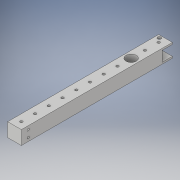
# Autodesk Inventor part: RobotArm Arm
Saved by Autodesk Inventor 2018 (Build 220112000, 112)
## iProperties
Created: 2018-01-13
Part Number: RobotArm Arm
Material: Generic
Document SubType Name: Modeling
Designer: lopez.xavier
Density: 1 g/cm^3
Appearance: Default
Author: lopez.xavier
Autodesk Inventor part; units mm, degrees
ref_plane "YZ Plane" through (0, 0, 0) normal (1, 0, 0) x (0, 1, 0)
ref_plane "XZ Plane" through (0, 0, 0) normal (0, 1, 0) x (-1, 0, 0)
ref_plane "XY Plane" through (0, 0, 0) normal (0, 0, 1) x (1, 0, 0)
sketch "Sketch1" plane through (0, 0, 0) normal (0, 0, 1) x (1, 0, 0)
  line L0 (0, 0) -> (279.4, 0)
  line L1 (279.4, 0) -> (279.4, 25.4)
  line L2 (279.4, 25.4) -> (0, 25.4)
  line L3 (0, 25.4) -> (0, 0)
  dimension "d0" = 279.4
  dimension "d1" = 25.4
  constraints: 8 end point, 2 parallel, 1 horizontal, 1 perpendicular
  measures "d0" distance of L2.end L1.end
  measures "d1" distance of L0.end L1.end
extrude "Extrusion1" add sketch "Sketch1" along normal blind 25.4
sketch "Sketch4" plane through (0, 0, 25.4) normal (0, 0, 1) x (1, 0, 0)
  circle A0 centre (12.7, 12.7) radius 2.3813
  line L0 (0, 0) -> (279.4, 0) projected
  line L1 (0, 25.4) -> (0, 0) projected
  circle A1 centre (38.1, 12.7) radius 2.3813
  circle A2 centre (63.5, 12.7) radius 2.3813
  circle A3 centre (88.9, 12.7) radius 2.3813
  circle A4 centre (114.3, 12.7) radius 2.3813
  circle A5 centre (139.7, 12.7) radius 2.3813
  circle A6 centre (165.1, 12.7) radius 2.3813
  circle A7 centre (190.5, 12.7) radius 2.3813
  circle A8 centre (215.9, 12.7) radius 2.3813
  circle A9 centre (241.3, 12.7) radius 2.3813
  circle A10 centre (266.7, 12.7) radius 2.3813
  circle A11 centre (292.1, 12.7) radius 2.3813
  circle A12 centre (317.5, 12.7) radius 2.3813
  circle A13 centre (63.5, 12.7) radius 9.525
  circle A14 centre (5.08, 6.35) radius 3.175
  dimension "d17" = 4.7625
  dimension "d18" = 12.7
  dimension "d19" = 12.7
  dimension "d22" = 25.4
  dimension "d37" = 19.05
  dimension "d46" = 6.35
  dimension "d48" = 6.35
  dimension "d49" = 58.42
  constraints: 15 centre point, 1 coincident, 1 horizontal, 24 other
  measures "d17" diameter of A0
  measures "d18" distance from line of L0 A0.centre
  measures "d19" distance from line of L1 A0.centre
  measures "d22" distance of A0.centre A1.centre
  measures "d37" diameter of A13
  measures "d46" diameter of A14
  measures "d48" distance from line of L0 A14.centre
  measures "d49" horizontal distance of A13.centre A14.centre
extrude "Extrusion4" cut sketch "Sketch4" against normal blind 25.4 contours A0 | A1 | A2 | A3 | A4 | A5 | A6 | A7 | A8 | A9 | A10 | A11 | A12 | A13 | A14
sketch "Sketch6" plane through (0, 25.4, 0) normal (0, 1, 0) x (1, 0, 0)
  line L0 (19.05, -22.225) -> (0, -22.225)
  line L1 (0, -22.225) -> (0, -3.175)
  line L2 (0, -3.175) -> (19.05, -3.175)
  line L3 (19.05, -3.175) -> (19.05, -22.225)
  line L4 (279.4, 0) -> (279.4, -25.4) projected
  line L5 (279.4, -25.4) -> (0, -25.4) projected
  line L6 (279.4, 0) -> (0, 0) projected
  line L7 (0, 0) -> (0, -25.4) projected
  dimension "d38" = 19.05
  dimension "d41" = 3.175
  dimension "d42" = 3.175
  dimension "d45" = 0
  constraints: 8 end point, 2 parallel, 1 horizontal, 1 perpendicular
  measures "d38" distance of L0.start L0.end
  measures "d41" distance between parallel lines of L5 L0
  measures "d42" distance between parallel lines of L6 L2
  measures "d45" distance between parallel lines of L7 L1
extrude "Extrusion6" cut sketch "Sketch6" against normal blind 25.4 contours L0 L1 L2 L3
sketch "Sketch7" plane through (0, 25.4, 0) normal (0, 1, 0) x (1, 0, 0)
  circle A0 centre (266.7, -18.9992) radius 2.0701
  circle A1 centre (266.7, -6.2992) radius 2.0701
  line L0 (279.4, 0) -> (279.4, -25.4) projected
  line L1 (279.4, 0) -> (0, 0) projected
  line L2 (279.4, -25.4) -> (0, -25.4) projected
  dimension "d50" = 4.1402
  dimension "d51" = 4.1402
  dimension "d52" = 12.7
  dimension "d53" = 12.7
  dimension "d54" = 12.7
  dimension "d58" = 6.4008
  constraints: 2 centre point
  measures "d50" diameter of A1
  measures "d51" diameter of A0
  measures "d52" distance of A1.centre A0.centre
  measures "d53" distance from line of L0 A0.centre
  measures "d54" distance from line of L0 A1.centre
  measures "d58" distance from line of L2 A0.centre
extrude "Extrusion7" cut sketch "Sketch7" against normal blind 25.4
equation "\"d42\" = d41"
equation "\"d51\" = d50"
equation "\"d53\" = d54"
body "Solid1"
